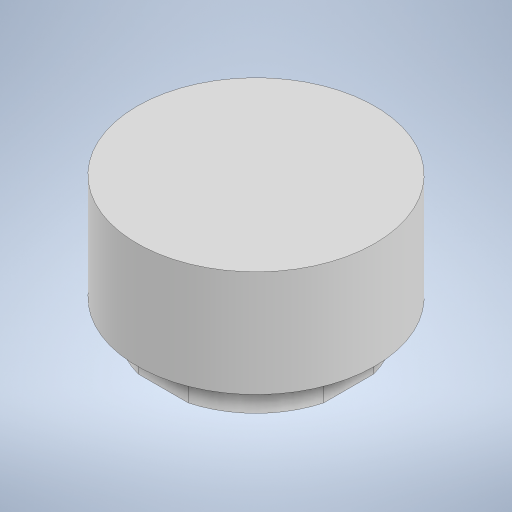
# Autodesk Inventor part: LED Assy
Saved by Autodesk Inventor 2024 (Build 280153020, 153B)
## iProperties
Created: 2023-08-04
Part Number: LED Assy
Material: Generic
Document SubType Name: Modeling
Designer: torban
Density: 1 g/cm^3
Appearance: Default
Author: torban
Autodesk Inventor part; units mm, degrees
ref_plane "YZ Plane" through (0, 0, 0) normal (1, 0, 0) x (0, 1, 0)
ref_plane "XZ Plane" through (0, 0, 0) normal (0, 1, 0) x (-1, 0, 0)
ref_plane "XY Plane" through (0, 0, 0) normal (0, 0, 1) x (1, 0, 0)
sketch "Sketch1" plane through (0, 0, 0) normal (0, 1, 0) x (-1, 0, 0)
  circle A0 centre (0, 0) radius 4.75
  dimension "d0" = 9.5
  constraints: 1 centre point, 1 coincident
  measures "d0" diameter of A0
extrude "Extrusion1" add sketch "Sketch1" along normal blind 1.6
sketch "Sketch2" plane through (0, 1.6, 0) normal (0, 1, 0) x (1, 0, 0)
  circle A0 centre (0, 0) radius 4.75 projected
  line L0 (2.5, -2.5) -> (-2.5, -2.5)
  line L1 (-2.5, -2.5) -> (-2.5, 2.5)
  line L2 (-2.5, 2.5) -> (2.5, 2.5)
  line L3 (2.5, 2.5) -> (2.5, -2.5)
  line L4 (2.5, -2.5) -> (-2.5, 2.5) construction
  line L5 (-2.5, -2.5) -> (2.5, 2.5) construction
  dimension "d3" = 5
  dimension "d4" = 5
  constraints: 12 end point, 2 midpoint, 2 parallel, 1 horizontal, 1 perpendicular
  measures "d3" distance of L1.end L2.end
  measures "d4" distance of L0.end L1.end
extrude "Extrusion2" add sketch "Sketch2" along normal blind 1.63 separate body contours L0 L1 L2 L3
sketch "Sketch3" plane through (0, 1.6, 0) normal (0, 1, 0) x (1, 0, 0)
  line L0 (-2.85, -1.1) -> (-3.85, -1.1)
  line L1 (-3.85, -1.1) -> (-3.85, 1.1)
  line L2 (-3.85, 1.1) -> (-2.85, 1.1)
  line L3 (-2.85, 1.1) -> (-2.85, -1.1)
  line L4 (-2.85, -1.1) -> (-3.85, 1.1) construction
  line L5 (-3.85, -1.1) -> (-2.85, 1.1) construction
  line L6 (3.85, -1.1) -> (2.85, -1.1)
  line L7 (2.85, -1.1) -> (2.85, 1.1)
  line L8 (2.85, 1.1) -> (3.85, 1.1)
  line L9 (3.85, 1.1) -> (3.85, -1.1)
  line L10 (3.85, -1.1) -> (2.85, 1.1) construction
  line L11 (2.85, -1.1) -> (3.85, 1.1) construction
  line L12 (-2.5, 2.5) -> (-2.5, -2.5) projected
  line L13 (-2.5, -2.5) -> (2.5, -2.5) projected
  line L14 (2.5, -2.5) -> (2.5, 2.5) projected
  point P0 (0, 0)
  point P1 (-3.35, 0)
  point P2 (3.35, 0)
  point P3 (-2.5, 0)
  dimension "d7" = 2.2
  dimension "d8" = 1
  dimension "d9" = 1
  dimension "d10" = 7.7
  dimension "d12" = 2.5
  dimension "d14" = 0.35
  dimension "d15" = 0.35
  constraints: 24 end point, 5 midpoint, 5 parallel, 2 horizontal, 2 perpendicular, 1 point on line
  measures "d7" distance of L0.end L1.end
  measures "d8" distance between parallel lines of L3 L1
  measures "d9" distance of L6.start L6.end
  measures "d10" distance between parallel lines of L9 L1
  measures "d12" distance from line of L13 point (-3.35, 0)
  measures "d14" distance from line of point (-2.5, 0) L3
  measures "d15" distance between parallel lines of L14 L7
extrude "Extrusion3" add sketch "Sketch3" along normal blind 0.5 separate body
sketch "Sketch4" plane through (0, 0, 0) normal (0, -1, 0) x (1, 0, 0)
  circle A0 centre (0, 0) radius 4.75 projected
  line L0 (-4.585, 4.585) -> (4.585, 4.585)
  line L1 (4.585, 4.585) -> (4.585, -4.585)
  line L2 (4.585, -4.585) -> (-4.585, -4.585)
  line L3 (-4.585, -4.585) -> (-4.585, 4.585)
  line L4 (-4.585, 4.585) -> (4.585, -4.585) construction
  line L5 (4.585, 4.585) -> (-4.585, -4.585) construction
  point P0 (1.2411, -4.585)
  point P1 (-1.2411, -4.585)
  point P2 (-1.2411, 4.585)
  point P3 (1.2411, 4.585)
  point P4 (-4.585, -1.2411)
  point P5 (-4.585, 1.2411)
  point P6 (4.585, 1.2411)
  point P7 (4.585, -1.2411)
  dimension "d18" = 9.17
  dimension "d19" = 9.17
  constraints: 12 end point, 2 midpoint, 2 parallel, 1 horizontal, 1 perpendicular
  measures "d18" distance of L1.end L2.end
  measures "d19" distance between parallel lines of L2 L0
extrude "Extrusion4" cut sketch "Sketch4" against normal through all contours A0 L1 | L0 A0 | A0 L2 | L3 A0 bodies 1
sketch "Sketch5" plane through (0, 0, 0) normal (0, -1, 0) x (1, 0, 0)
  line L0 (1.2411, 4.585) -> (-1.2411, 4.585) projected
  line L1 (0, 4.585) -> (0, -4.585) construction
  line L2 (-1.2411, -4.585) -> (1.2411, -4.585) projected
  line L3 (-4.585, 1.2411) -> (-4.585, -1.2411) projected
  line L4 (-4.585, 0) -> (4.585, 0) construction
  line L5 (4.585, -1.2411) -> (4.585, 1.2411) projected
  line L6 (-2.5, -2.5) -> (-2.5, 2.5) projected
  line L7 (0, 2.435) -> (0, 1.605) construction
  line L8 (-0.75, 2.435) -> (-0.75, 1.605)
  line L9 (0.75, 1.605) -> (0.75, 2.435)
  arc A0 (0.75, 2.435) -> (-0.75, 2.435) centre (0, 2.435) ccw
  arc A1 (-0.75, 1.605) -> (0.75, 1.605) centre (0, 1.605) ccw
  line L10 (0, -4.585) -> (0, 4.585) construction
  line L11 (0, -2.435) -> (0, -1.605) construction
  line L12 (-0.75, -2.435) -> (-0.75, -1.605)
  line L13 (0.75, -1.605) -> (0.75, -2.435)
  arc A2 (-0.75, -2.435) -> (0.75, -2.435) centre (0, -2.435) ccw
  arc A3 (0.75, -1.605) -> (-0.75, -1.605) centre (0, -1.605) ccw
  line L14 (-3.25, 2.435) -> (-3.25, 1.605)
  line L15 (-2.5, 2.435) -> (-2.5, 1.605) construction
  arc A4 (-3.25, 1.605) -> (-1.75, 1.605) centre (-2.5, 1.605) ccw
  line L16 (-1.75, 1.605) -> (-1.75, 2.435)
  arc A5 (-1.75, 2.435) -> (-3.25, 2.435) centre (-2.5, 2.435) ccw
  line L17 (-2.5, 4.585) -> (-2.5, -4.585) construction
  line L18 (-2.5, -4.585) -> (-2.5, 4.585) construction
  arc A6 (-3.25, -2.435) -> (-1.75, -2.435) centre (-2.5, -2.435) ccw
  line L19 (-2.5, -2.435) -> (-2.5, -1.605) construction
  line L20 (-3.25, -2.435) -> (-3.25, -1.605)
  line L21 (-1.75, -1.605) -> (-1.75, -2.435)
  arc A7 (-1.75, -1.605) -> (-3.25, -1.605) centre (-2.5, -1.605) ccw
  line L22 (1.75, 2.435) -> (1.75, 1.605)
  line L23 (2.5, 2.435) -> (2.5, 1.605) construction
  arc A8 (1.75, 1.605) -> (3.25, 1.605) centre (2.5, 1.605) ccw
  line L24 (3.25, 1.605) -> (3.25, 2.435)
  arc A9 (3.25, 2.435) -> (1.75, 2.435) centre (2.5, 2.435) ccw
  line L25 (2.5, 4.585) -> (2.5, -4.585) construction
  line L26 (2.5, -4.585) -> (2.5, 4.585) construction
  arc A10 (1.75, -2.435) -> (3.25, -2.435) centre (2.5, -2.435) ccw
  line L27 (2.5, -2.435) -> (2.5, -1.605) construction
  line L28 (1.75, -2.435) -> (1.75, -1.605)
  line L29 (3.25, -1.605) -> (3.25, -2.435)
  arc A11 (3.25, -1.605) -> (1.75, -1.605) centre (2.5, -1.605) ccw
  line L30 (-0.75, 2.435) -> (-0.75, 1.605)
  line L31 (0, 2.435) -> (0, 1.605) construction
  arc A12 (-0.75, 1.605) -> (0.75, 1.605) centre (0, 1.605) ccw
  line L32 (0.75, 1.605) -> (0.75, 2.435)
  arc A13 (0.75, 2.435) -> (-0.75, 2.435) centre (0, 2.435) ccw
  line L33 (0, 4.585) -> (0, -4.585) construction
  line L34 (0, -4.585) -> (0, 4.585) construction
  arc A14 (-0.75, -2.435) -> (0.75, -2.435) centre (0, -2.435) ccw
  line L35 (0, -2.435) -> (0, -1.605) construction
  line L36 (-0.75, -2.435) -> (-0.75, -1.605)
  line L37 (0.75, -1.605) -> (0.75, -2.435)
  arc A15 (0.75, -1.605) -> (-0.75, -1.605) centre (0, -1.605) ccw
  point P0 (0, 0)
  point P1 (0, 2.02)
  point P2 (-0.75, 2.02)
  point P3 (0, 0.855)
  point P4 (0, 3.185)
  point P5 (0, -2.02)
  point P6 (-0.75, -2.02)
  point P7 (0, -0.855)
  point P8 (0, -3.185)
  point P9 (0, -0.855)
  point P10 (-3.25, 2.02)
  point P11 (-2.5, 0.855)
  point P12 (-2.5, 2.02)
  point P13 (-2.5, 3.185)
  point P14 (-2.5, -2.02)
  point P15 (-2.5, -3.185)
  point P16 (-2.5, -0.855)
  point P17 (-2.5, -0.855)
  point P18 (-3.25, -2.02)
  point P19 (1.75, 2.02)
  point P20 (2.5, 0.855)
  point P21 (2.5, 2.02)
  point P22 (2.5, 3.185)
  point P23 (2.5, -2.02)
  point P24 (2.5, -3.185)
  point P25 (2.5, -0.855)
  point P26 (2.5, -0.855)
  point P27 (1.75, -2.02)
  point P28 (-0.75, 2.02)
  point P29 (0, 0.855)
  point P30 (0, 2.02)
  point P31 (0, 3.185)
  point P32 (0, -2.02)
  point P33 (0, -3.185)
  point P34 (0, -0.855)
  point P35 (0, -0.855)
  point P36 (-0.75, -2.02)
  dimension "d24" = 1.5
  dimension "d25" = 2.33
  dimension "d26" = 1.4
  dimension "d27" = 1.71
  dimension "d30" = 2.5
  dimension "d33" = 2.5
  constraints: 82 end point, 35 point on circle, 16 centre point, 12 symmetric about line, 8 point on line, 6 midpoint, 4 tangent, 2 horizontal, 1 parallel, 1 vertical, 113 other
  measures "d24" distance from line of point (-0.75, 2.02) L9
  measures "d25" distance of point (0, 0.855) point (0, 3.185)
  measures "d26" distance from line of L0 point (0, 3.185)
  measures "d27" distance of point (0, -0.855) point (0, 0.855)
  measures "d30" distance of L8.end L14.end
  measures "d33" distance of L8.end L22.end
extrude "Extrusion5" add sketch "Sketch5" along normal blind 0.1 separate body
sketch "Sketch6" plane through (0, 1.6, 0) normal (0, 1, 0) x (1, 0, 0)
  line L0 (4.585, 1.2411) -> (4.585, -1.2411) projected
  arc A0 (1.2411, -4.585) -> (4.585, -1.2411) centre (0, 0) ccw projected
  line L1 (1.2411, -4.585) -> (-1.2411, -4.585) projected
  arc A1 (-4.585, -1.2411) -> (-1.2411, -4.585) centre (0, 0) ccw projected
  line L2 (-4.585, -1.2411) -> (-4.585, 1.2411) projected
  arc A2 (-1.2411, 4.585) -> (-4.585, 1.2411) centre (0, 0) ccw projected
  line L3 (-1.2411, 4.585) -> (1.2411, 4.585) projected
  arc A3 (4.585, 1.2411) -> (1.2411, 4.585) centre (0, 0) ccw projected
  line L4 (2.5, 2.5) -> (2.5, -2.5) projected
  line L5 (2.5, -2.5) -> (-2.5, -2.5) projected
  line L6 (-2.5, -2.5) -> (-2.5, 2.5) projected
  line L7 (-2.5, 2.5) -> (2.5, 2.5) projected
  line L8 (-2.85, 1.1) -> (-2.85, -1.1) projected
  line L9 (-2.85, -1.1) -> (-3.85, -1.1) projected
  line L10 (-3.85, -1.1) -> (-3.85, 1.1) projected
  line L11 (-3.85, 1.1) -> (-2.85, 1.1) projected
  line L12 (3.85, 1.1) -> (3.85, -1.1) projected
  line L13 (3.85, -1.1) -> (2.85, -1.1) projected
  line L14 (2.85, -1.1) -> (2.85, 1.1) projected
  line L15 (2.85, 1.1) -> (3.85, 1.1) projected
  line L16 (1.3059, 5.085) -> (-1.3059, 5.085)
  arc A4 (-1.3059, 5.085) -> (-5.085, 1.3059) centre (0, 0) ccw
  line L17 (-5.085, 1.3059) -> (-5.085, -1.3059)
  arc A5 (-5.085, -1.3059) -> (-1.3059, -5.085) centre (0, 0) ccw
  line L18 (-1.3059, -5.085) -> (1.3059, -5.085)
  arc A6 (1.3059, -5.085) -> (5.085, -1.3059) centre (0, 0) ccw
  line L19 (5.085, -1.3059) -> (5.085, 1.3059)
  arc A7 (5.085, 1.3059) -> (1.3059, 5.085) centre (0, 0) ccw
  line L20 (-4.385, 1.2142) -> (-4.385, -1.2142)
  arc A8 (-4.385, -1.2142) -> (-1.2142, -4.385) centre (0, 0) ccw
  line L21 (-1.2142, -4.385) -> (1.2142, -4.385)
  arc A9 (1.2142, -4.385) -> (4.385, -1.2142) centre (0, 0) ccw
  line L22 (4.385, -1.2142) -> (4.385, 1.2142)
  arc A10 (4.385, 1.2142) -> (1.2142, 4.385) centre (0, 0) ccw
  line L23 (1.2142, 4.385) -> (-1.2142, 4.385)
  arc A11 (-1.2142, 4.385) -> (-4.385, 1.2142) centre (0, 0) ccw
  line L24 (3, 3) -> (3, -3)
  line L25 (3.4209, -3) -> (-3.4209, -3)
  line L26 (-3, -3) -> (-3, 3)
  line L27 (-3.4209, 3) -> (3.4209, 3)
  dimension "d38" = 0.5
  dimension "d39" = 0.2
  dimension "d40" = 0.5
  constraints: 24 end point, 20 point on circle, 8 centre point, 4 point on line, 14 other
  measures "d38" distance between parallel lines of L3 L16
  measures "d39" radial gap between concentric circles of A2 A11
  measures "d40" distance between parallel lines of L7 L27
extrude "Extrusion6" add sketch "Sketch6" along normal blind 1.75 separate body contours L0 A0 L1 A1 L2 A2 L3 A3 | L27 A11 L23 A10 | L25 A9 L21 A8 | A7 L19 A6 L18 A5 L17 A4 L16
sketch "Sketch7" plane through (0, 3.35, 0) normal (0, 1, 0) x (1, 0, 0)
  arc A0 (-4.385, -1.2142) -> (-3.4209, -3) centre (0, 0) ccw projected
  line L0 (-3.4209, -3) -> (3.4209, -3) projected
  arc A1 (3.4209, -3) -> (4.385, -1.2142) centre (0, 0) ccw projected
  line L1 (4.385, -1.2142) -> (4.385, 1.2142) projected
  arc A2 (4.385, 1.2142) -> (3.4209, 3) centre (0, 0) ccw projected
  line L2 (3.4209, 3) -> (-3.4209, 3) projected
  arc A3 (-3.4209, 3) -> (-4.385, 1.2142) centre (0, 0) ccw projected
  line L3 (-4.385, 1.2142) -> (-4.385, -1.2142) projected
  line L4 (-1.3059, 5.085) -> (1.3059, 5.085) projected
  arc A4 (5.085, 1.3059) -> (1.3059, 5.085) centre (0, 0) ccw projected
  line L5 (5.085, 1.3059) -> (5.085, -1.3059) projected
  arc A5 (1.3059, -5.085) -> (5.085, -1.3059) centre (0, 0) ccw projected
  line L6 (1.3059, -5.085) -> (-1.3059, -5.085) projected
  arc A6 (-5.085, -1.3059) -> (-1.3059, -5.085) centre (0, 0) ccw projected
  line L7 (-5.085, -1.3059) -> (-5.085, 1.3059) projected
  arc A7 (-1.3059, 5.085) -> (-5.085, 1.3059) centre (0, 0) ccw projected
  circle A8 centre (0, 0) radius 5.875
  dimension "d43" = 11.75
  constraints: 1 centre point, 1 coincident
  measures "d43" diameter of A8
extrude "Extrusion7" add sketch "Sketch7" against normal up to surface (1.75 mm away) contours L4 A4 L5 A5 L6 A6 L7 A7 | A8 bodies 5
sketch "Sketch8" plane through (0, 3.35, 0) normal (0, 1, 0) x (1, 0, 0)
  circle A0 centre (0, 0) radius 5.875 projected
  arc A1 (-4.385, -1.2142) -> (-3.4209, -3) centre (0, 0) ccw projected
  line L0 (-3.4209, -3) -> (3.4209, -3) projected
  arc A2 (3.4209, -3) -> (4.385, -1.2142) centre (0, 0) ccw projected
  line L1 (4.385, -1.2142) -> (4.385, 1.2142) projected
  arc A3 (4.385, 1.2142) -> (3.4209, 3) centre (0, 0) ccw projected
  line L2 (3.4209, 3) -> (-3.4209, 3) projected
  arc A4 (-3.4209, 3) -> (-4.385, 1.2142) centre (0, 0) ccw projected
  line L3 (-4.385, 1.2142) -> (-4.385, -1.2142) projected
extrude "Extrusion8" add sketch "Sketch8" along normal blind 3.5 contours A0 | L3 A4 L2 A3 L1 A2 L0 A1 bodies 5
equation "\"d9\" = d8"
equation "\"d15\" = d14"
equation "\"d19\" = d18"
